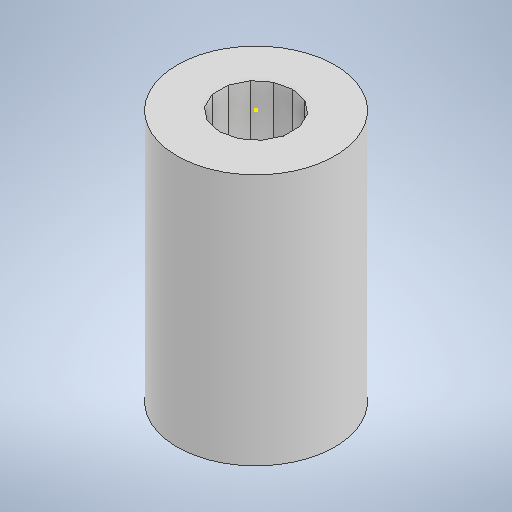
# Autodesk Inventor part: spool_motor
Saved by Autodesk Inventor 2025.2 (Build 292293000, 293)
## iProperties
Created: 2024-12-25
Part Number: spool_motor
Material: Ogólny
Document SubType Name: Modeling
Designer: Mos
Density: 1 g/cm^3
Appearance: Domyślna
Author: Mos
Autodesk Inventor part; units mm, degrees
ref_plane "YZ Plane" through (0, 0, 0) normal (1, 0, 0) x (0, 1, 0)
ref_plane "XZ Plane" through (0, 0, 0) normal (0, 1, 0) x (-1, 0, 0)
ref_plane "XY Plane" through (0, 0, 0) normal (0, 0, 1) x (1, 0, 0)
sketch "Szkic1" plane through (0, 0, 0) normal (0, 1, 0) x (-1, 0, 0)
  circle A0 centre (0, 0) radius 9.915
  constraints: 1 centre point, 1 coincident
extrude "Wyciągnięcie proste1" add sketch "Szkic1" along normal blind 31.7
sketch "Szkic2" plane through (0, 31.7, 0) normal (0, 1, 0) x (1, 0, 0)
  point P0 (0, 0)
sketch "Szkic3" plane through (0, 31.7, 0) normal (0, 1, 0) x (1, 0, 0)
  point P0 (0, 0)
sketch "Szkic4" plane through (0, 31.7, 0) normal (0, 1, 0) x (1, 0, 0)
  line L0 (4.499, -1.0269) -> (3.6079, -2.8772)
  line L1 (3.6079, -2.8772) -> (2.0022, -4.1577)
  line L2 (2.0022, -4.1577) -> (0, -4.6147)
  line L3 (0, -4.6147) -> (-2.0022, -4.1577)
  line L4 (-2.0022, -4.1577) -> (-3.6079, -2.8772)
  line L5 (-3.6079, -2.8772) -> (-4.499, -1.0269)
  line L6 (-4.499, -1.0269) -> (-4.499, 1.0269)
  line L7 (-4.499, 1.0269) -> (-3.6079, 2.8772)
  line L8 (-3.6079, 2.8772) -> (-2.0022, 4.1577)
  line L9 (-2.0022, 4.1577) -> (0, 4.6147)
  line L10 (0, 4.6147) -> (2.0022, 4.1577)
  line L11 (2.0022, 4.1577) -> (3.6079, 2.8772)
  line L12 (3.6079, 2.8772) -> (4.499, 1.0269)
  line L13 (4.499, 1.0269) -> (4.499, -1.0269)
  point P0 (0, 0)
  point P1 (0, 0)
  dimension "d2" = 4.6147
  constraints: 28 end point, 1 coincident, 29 other
  measures "d2" distance of L12.end point (0, 0)
extrude "Wyciągnięcie proste2" cut sketch "Szkic4" against normal blind 40
